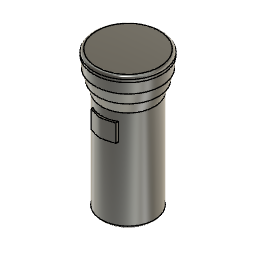
lanterna led v1 (Autodesk Fusion 360 design; units mm, degrees)
Autodesk Fusion 360 part; units mm, degrees
sketch "Sketch1" plane through (0, 0, 0) normal (0, 1, 0) x (1, 0, 0)
sketch "Sketch2" plane through (0, 0, 0) normal (0, 0, 1) x (1, 0, 0)
  circle A0 centre (0, 0) radius 25
  dimension "d1" = 50
  constraint coincident A0.centre origin
  measures "d1" diameter of A0
extrude "Extrude1" add sketch "Sketch2" along normal blind 75 makes body 1
extrude "Extrude2" add 1 faces at (2.6796, -11.7401, 75) along direction (0, 0, 1) blind 10 draft 20 on bodies 1 bodies 1
extrude "Extrude3" add 1 faces at (-16.6777, 5.9855, 85) along direction (0, 0, 1) blind 10 draft 15 on bodies 1 bodies 1
extrude "Extrude4" add 1 faces at (6.1371, -15.1267, 95) along direction (0, 0, 1) blind 10 draft 5 on bodies 1 bodies 1
extrude "Extrude5" add 1 faces at (4.1899, -7.8193, 105) along direction (0, 0, 1) blind 5 on bodies 1 bodies 1
fillet "Fillet1" radius 2.5 1 edges at (-30.0154, -11.6419, 110) on bodies 1
extrude "Extrude6" add 1 faces at (2.6796, -11.7401, 0) along direction (0, 0, -1) blind 10 on bodies 1 bodies 1
extrude "Extrude7" add 1 faces at (2.6796, -11.7401, -10) along direction (0, 0, -1) blind 10 on bodies 1 bodies 1
fillet "Fillet2" radius 2 1 edges at (-23.3082, 9.0404, -20) on bodies 1
sketch "Sketch3" plane through (0, 0, 0) normal (0, 1, 0) x (1, 0, 0)
  line L0 (-8.8325, -65.1718, -25) -> (10.3177, -65.1718, -25)
  line L1 (10.3177, -65.1718, -25) -> (10.3177, -52.825, -25)
  line L2 (10.3177, -52.825, -25) -> (-8.8325, -52.825, -25)
  line L3 (-8.8325, -52.825, -25) -> (-8.8325, -65.1718, -25)
extrude "Extrude8" cut sketch "Sketch3" along normal blind 5 contours L0 L1 L2 L3 in plane through (0, -25, 0) normal (0, 1, 0) bodies 1
sketch "Sketch4" plane through (0, -20, 0) normal (0, -1, 0) x (1, 0, 0)
  line L0 (-8.8325, 65.1718) -> (-8.8325, 52.825)
  line L1 (-8.8325, 52.825) -> (10.3177, 52.825)
  line L2 (10.3177, 52.825) -> (10.3177, 65.1718)
  line L3 (10.3177, 65.1718) -> (-8.8325, 65.1718)
  line L4 (-11.0318, 50.6256) -> (12.517, 50.6256)
  line L5 (12.517, 50.6256) -> (12.517, 67.3711)
  line L6 (12.517, 67.3711) -> (-11.0318, 67.3711)
  line L7 (-11.0318, 67.3711) -> (-11.0318, 50.6256)
  dimension "d22" = 2.1993
extrude "Extrude9" cut sketch "Sketch4" along normal blind 32 bodies 1
extrude "Extrude10" add 1 faces at (-3.1822, -20, 56.2075) along direction (0, -1, 0) blind 8 separate body on bodies 1 makes body 2
sketch "Sketch5" plane through (0, 0, 50.6256) normal (0, 0, -1) x (1, 0, 0)
  line L0 (-11.0318, 20) -> (12.517, 20)
  line L1 (12.517, 20) -> (12.517, 28)
  line L2 (12.517, 28) -> (-11.0318, 28)
  line L3 (-11.0318, 28) -> (-11.0318, 20)
  spline S0 degree 2 poles (-11.0318, 24) (0.1748, 28) (12.517, 24) knots 0 0 0 2.430212 2.430212 2.430212 weights 1 3 1
  constraint midpoint L1 S0.end
  constraint midpoint L3 S0.start
extrude "Extrude11" cut sketch "Sketch5" against normal blind 17 contours L1 L2 L3 S0 bodies 2
